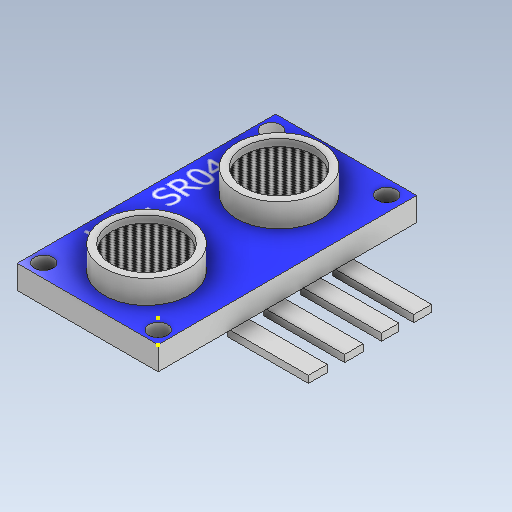
# Autodesk Inventor part: ultrasonic now
Saved by Autodesk Inventor 2021 (Build 250183000, 183)
## iProperties
Created: 2021-07-14
Part Number: ultrasonic now
Material: Generic
Document SubType Name: Modeling
Designer: Dell
Density: 1 g/cm^3
Appearance: Default
Author: Dell
Autodesk Inventor part; units mm, degrees
ref_plane "YZ Plane" through (0, 0, 0) normal (1, 0, 0) x (0, 1, 0)
ref_plane "XZ Plane" through (0, 0, 0) normal (0, 1, 0) x (-1, 0, 0)
ref_plane "XY Plane" through (0, 0, 0) normal (0, 0, 1) x (1, 0, 0)
sketch "Sketch1" plane through (0, 0, 0) normal (0, 1, 0) x (-1, 0, 0)
  line L0 (0, 0) -> (60, 0)
  line L1 (60, 0) -> (60, -110)
  line L2 (60, -110) -> (0, -110)
  line L3 (0, -110) -> (0, 0)
  dimension "d0" = 110
  dimension "d1" = 60
  constraints: 8 end point, 2 parallel, 1 horizontal, 1 perpendicular
  measures "d0" distance of L0.end L1.end
  measures "d1" distance of L1.end L2.end
sketch "Sketch2" plane through (0, 0, 0) normal (0, 1, 0) x (-1, 0, 0)
  line L0 (1.1114, -30.6908) -> (-33.2555, -30.6908)
  line L1 (-33.2555, -30.6908) -> (-33.2555, -38.7269)
  line L2 (-33.2555, -38.7269) -> (1.1114, -38.7269)
  line L3 (1.1114, -38.7269) -> (1.1114, -30.6908)
  line L4 (1.1114, -46.079) -> (-33.2555, -46.079)
  line L5 (-33.2555, -46.079) -> (-33.2555, -53.9441)
  line L6 (-33.2555, -53.9441) -> (1.1114, -53.9441)
  line L7 (1.1114, -53.9441) -> (1.1114, -46.079)
  line L8 (1.1114, -61.8091) -> (-33.2555, -61.8091)
  line L9 (-33.2555, -61.8091) -> (-33.2555, -69.1613)
  line L10 (-33.2555, -69.1613) -> (1.1114, -69.1613)
  line L11 (1.1114, -69.1613) -> (1.1114, -61.8091)
  line L12 (1.1114, -75.4875) -> (-33.2555, -75.4875)
  line L13 (-33.2555, -75.4875) -> (-33.2555, -83.0106)
  line L14 (-33.2555, -83.0106) -> (1.1114, -83.0106)
  line L15 (1.1114, -83.0106) -> (1.1114, -75.4875)
  point P0 (0, 0)
  constraints: 32 end point, 8 parallel, 6 point on line, 4 horizontal, 4 perpendicular
extrude "Extrusion1" add sketch "Sketch1" along normal blind 10
extrude "Extrusion2" add sketch "Sketch2" against normal blind 3
sketch "Sketch3" plane through (0, 10, 0) normal (0, 1, 0) x (1, 0, 0)
  circle A0 centre (-29.665, 24.7066) radius 18.0252
  circle A1 centre (-29.665, 81.1298) radius 18.0284
  point P0 (0, 0)
  constraints: 2 centre point
extrude "Extrusion3" add sketch "Sketch3" along normal blind 10
sketch "Sketch4" plane through (-29.665, 20, -24.7066) normal (0, 1, 0) x (1, 0, 0)
  point P0 (29.665, -24.7066)
sketch "Sketch5" plane through (-29.665, 20, -24.7066) normal (0, 1, 0) x (1, 0, 0)
  circle A0 centre (0, 0) radius 18.0252 projected
  point P0 (29.665, -24.7066)
  constraints: 1 coincident
hole "Hole1" at (-29.665, 20, -24.7066) direction (0, -1, 0) diameter 30 depth 3
sketch "Sketch6" plane through (-29.665, 20, -81.1298) normal (0, 1, 0) x (1, 0, 0)
  circle A0 centre (0, 0) radius 18.0284 projected
  point P0 (29.665, -81.1298)
  constraints: 1 coincident
hole "Hole2" at (-29.665, 20, -81.1298) direction (0, -1, 0) diameter 30 depth 3
sketch "Sketch7" plane through (0, 10, 0) normal (0, 1, 0) x (1, 0, 0)
  point P0 (0, 0)
  point P1 (-54.5256, 5.8465)
  point P2 (-54.9391, 103.1409)
  point P3 (-6.5559, 103.7715)
  point P4 (-5.4452, 5.4602)
hole "Hole3" at (-54.5256, 10, -5.8465) at (-54.9391, 10, -103.1409) at (-6.5559, 10, -103.7715) at (-5.4452, 10, -5.4602) direction (0, -1, 0) diameter 8 end through all
sketch "Sketch8" plane through (0, 10, 0) normal (0, 1, 0) x (1, 0, 0)
  line L0 (-57.5346, 24.8775) -> (-57.5346, 80.9707) construction
  line L1 (-57.5346, 80.9707) -> (-48.1627, 80.9707) construction
  line L2 (-48.1627, 80.9707) -> (-48.1627, 24.8775) construction
  line L3 (-48.1627, 24.8775) -> (-57.5346, 24.8775) construction
  point P0 (0, 0)
  constraints: 2 other
body "Solid1"
